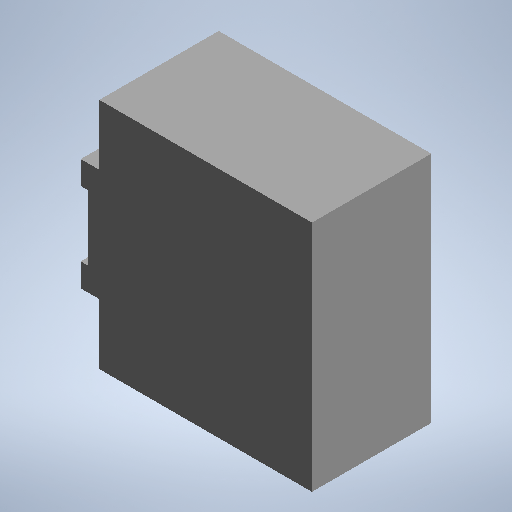
# Autodesk Inventor part: MW_WDR_240_24
Saved by Autodesk Inventor 2025.4 (Build 294407000, 407)
## iProperties
Created: 2026-07-01
Part Number: MW_WDR_240_24
Material: Générique
Document SubType Name: Modeling
Designer: louis
Density: 1 g/cm^3
Appearance: Par défaut
Author: louis
Autodesk Inventor part; units mm, degrees
ref_plane "YZ Plane" through (0, 0, 0) normal (1, 0, 0) x (0, 1, 0)
ref_plane "XZ Plane" through (0, 0, 0) normal (0, 1, 0) x (-1, 0, 0)
ref_plane "XY Plane" through (0, 0, 0) normal (0, 0, 1) x (1, 0, 0)
sketch "Sketch2" plane through (0, 0, 0) normal (0, 1, 0) x (-1, 0, 0)
  line L0 (57, -62.5) -> (-57, -62.5)
  line L1 (-57, -62.5) -> (-57, 62.5)
  line L2 (-57, 62.5) -> (57, 62.5)
  line L3 (57, 62.5) -> (57, -62.5)
  line L4 (57, -62.5) -> (-57, 62.5) construction
  line L5 (-57, -62.5) -> (57, 62.5) construction
  line L6 (57, 30) -> (57, -30)
  line L7 (57, -30) -> (67, -30)
  line L8 (67, -30) -> (67, 30)
  line L9 (67, 30) -> (57, 30)
  line L10 (67, 17.5) -> (67, -17.5)
  line L11 (67, -17.5) -> (63, -17.5)
  line L12 (63, -17.5) -> (63, 17.5)
  line L13 (63, 17.5) -> (67, 17.5)
  line L14 (63, 0) -> (57, 0) construction
  line L15 (67, 0) -> (57, 0) construction
  line L16 (67, 0) -> (57, 0) construction
  point P0 (0, 0)
  dimension "d0" = 114
  dimension "d1" = 125
  dimension "d2" = 6
  dimension "d3" = 10
  dimension "d4" = 35
  dimension "d5" = 60
  dimension "d6" = 12.5
  constraints: 34 end point, 8 midpoint, 6 parallel, 4 horizontal, 4 point on line, 3 perpendicular
  measures "d0" distance of L1.end L2.end
  measures "d1" distance of L0.end L1.end
  measures "d2" distance between parallel lines of L3 L12
  measures "d3" distance between parallel lines of L8 L3
  measures "d4" distance of L11.end L12.end
  measures "d5" distance of L6.start L6.end
  measures "d6" distance from line of L10.start L9
extrude "Extrusion1" add sketch "Sketch2" along normal mid plane 64 contours L0 L1 L2 L3 | L3 L9 L8 L13 L12 L11 L7
body "Solid1"
